Autodesk Fusion 360 part; units mm, degrees
note: some values were not read from the file. Chosen so that the rebuilt part matches the saved one: which bodies a step acts on. Set by a fixed rule: which sketch regions a step uses.
(part 2 of 2)
extrude "Extrude3" add sketch "Sketch1" along normal blind 6.7 contours L0 L1 L2 L3 L4 L5 A0 A1 A2 A3 A4 A5 bodies 1
extrude "Extrude5" add sketch "Sketch2" along normal blind 2 separate body contours A0 L0 L1 A80 A159 | A1 L2 L3 A80 A159 | A2 L4 L5 A81 A120 | A3 L6 L7 A81 A120 | A4 L8 L9 A82 A121 | A5 L10 L11 A82 A121 | A6 L12 L13 A83 A122 | A7 L14 L15 A83 A122 | A8 L16 L17 A84 A135 | A9 L18 L19 A84 A135 | A10 L20 L21 A85 A131 | A11 L22 L23 A85 A131 | A12 L24 L25 A86 A127 | A13 L26 L27 A86 A127 | A14 L28 L29 A87 A123 | A15 L30 L31 A87 A123 | A16 L32 L33 A88 A158 | A17 L34 L35 A88 A158 | A18 L36 L37 A89 A132 | A19 L38 L39 A89 A132 | A20 L40 L41 A90 A128 | A21 L42 L43 A90 A128 | A22 L44 L45 A91 A124 | A23 L46 L47 A91 A124 | A24 L48 L49 A92 A136 | A25 L50 L51 A92 A136 | A26 L52 L53 A93 A133 | A27 L54 L55 A93 A133 | A28 L56 L57 A94 A129 | A29 L58 L59 A94 A129 | A30 L60 L61 A95 A125 | A31 L62 L63 A95 A125 | A32 L64 L65 A96 A137 | A33 L66 L67 A96 A137 | A34 L68 L69 A97 A134 | A35 L70 L71 A97 A134 | A36 L72 L73 A98 A130 | A37 L74 L75 A98 A130 | A38 L76 L77 A99 A126 | A39 L78 L79 A99 A126 | A40 L80 L81 A100 A157 | A41 L82 L83 A100 A157 | A42 L84 L85 A101 A152 | A43 L86 L87 A101 A152 | A44 L88 L89 A102 A147 | A45 L90 L91 A102 A147 | A46 L92 L93 A103 A142 | A47 L94 L95 A103 A142 | A48 L96 L97 A104 A156 | A49 L98 L99 A104 A156 | A50 L100 L101 A105 A151 | A51 L102 L103 A105 A151 | A52 L104 L105 A106 A146 | A53 L106 L107 A106 A146 | A54 L108 L109 A107 A141 | A55 L110 L111 A107 A141 | A56 L112 L113 A108 A155 | A57 L114 L115 A108 A155 | A58 L116 L117 A109 A150 | A59 L118 L119 A109 A150 | A60 L120 L121 A110 A145 | A61 L122 L123 A110 A145 | A62 L124 L125 A111 A140 | A63 L126 L127 A111 A140 | A64 L128 L129 A112 A154 | A65 L130 L131 A112 A154 | A66 L132 L133 A113 A149 | A67 L134 L135 A113 A149 | A68 L136 L137 A114 A144 | A69 L138 L139 A114 A144 | A70 L140 L141 A115 A139 | A71 L142 L143 A115 A139 | A72 L144 L145 A116 A153 | A73 L146 L147 A116 A153 | A74 L148 L149 A117 A148 | A75 L150 L151 A117 A148 | A76 L152 L153 A118 A143 | A77 L154 L155 A118 A143 | A78 L156 L157 A119 A138 | A79 L158 L159 A119 A138 makes body 10 at (4.262, 7.3818, 0.6667) makes body 11 at (11.2811, -4.9625, 1.3333) makes body 12 at (-2.5256, 2.4663, 0.6667) makes body 13 at (12.115, 11.6015, 1.3333) makes body 14 at (22.5458, -5.5564, 0.6667) makes body 15 at (39.4227, -3.4161, 1.3333) makes body 16 at (33.1565, 1.6483, 1.3333) makes body 17 at (45.7149, 10.6668, 0.6667) makes body 18 at (16.2993, 19.8547, 1.3333) makes body 19 at (2.6839, 32.0105, 0.6667) makes body 20 at (27.8838, 27.9663, 1.3333) makes body 21 at (45.5449, 15.0482, 1.3333) makes body 22 at (12.7906, 14.4698, 1.3333) makes body 23 at (7.735, 27.078, 0.6667) makes body 24 at (21.9274, 24.1763, 1.3333) makes body 25 at (47.1273, 20.132, 0.6667) makes body 26 at (76.8247, -8.3362, 1.3333) makes body 27 at (96.5209, -4.8632, 1.3333) makes body 28 at (104.6325, 6.7213, 1.3333) makes body 29 at (84.0972, 9.8134, 1.3333) makes body 30 at (63.9057, 6.419, 1.3333) makes body 31 at (73.1464, 17.7127, 1.3333) makes body 32 at (89.7711, 21.0864, 1.3333) makes body 33 at (98.7218, 26.1059, 1.3333) makes body 34 at (80.6243, 29.5096, 1.3333) makes body 35 at (69.1776, 20.8965, 1.3333) makes body 36 at (71.4099, 27.5608, 1.3333) makes body 37 at (90.4723, 31.2461, 1.3333) makes body 38 at (101.0599, 23.2206, 1.3333) makes body 39 at (83.7119, 19.0225, 1.3333) makes body 40 at (62.6646, 16.1885, 1.3333) makes body 41 at (72.2711, 7.966, 1.3333) makes body 42 at (94.4246, 11.4019, 1.3333) makes body 43 at (106.369, -3.1267, 1.3333) makes body 44 at (86.6728, -6.5997, 1.3333) makes body 45 at (66.6168, -3.6556, 1.3333) makes body 46 at (32.8778, 27.3251, 1.3333) makes body 47 at (16.5459, 31.0086, 1.3333) makes body 48 at (4.4927, 23.0757, 1.3333) makes body 49 at (25.8487, 18.5212, 1.3333) makes body 50 at (17.5831, 25.3415, 0.6667) makes body 51 at (0.4947, 17.8012, 1.3333) makes body 52 at (22.1494, 12.8437, 1.3333) makes body 53 at (33.5476, 17.9766, 1.3333) makes body 54 at (41.3264, 6.4266, 1.3333) makes body 55 at (32.3297, -3.041, 1.3333) makes body 56 at (21.235, 2.8507, 1.3333) makes body 57 at (4.7147, 11.7431, 1.3333) makes body 58 at (8.415, 1.4895, 1.3333) makes body 59 at (2.1505, -2.7993, 1.3333) makes body 60 at (11.8885, 4.5947, 0.6667) makes body 61 at (18.2631, -0.2469, 1.3333) makes body 62 at (41.2681, -9.9363, 1.3333) makes body 63 at (32.7691, 7.8395, 1.3333) makes body 64 at (84.9363, 3.2484, 1.3333) makes body 65 at (65.2402, -0.2246, 1.3333) makes body 66 at (73.3518, 11.36, 1.3333) makes body 67 at (90.6102, 14.5214, 1.3333) makes body 68 at (100.3204, 32.9825, 1.3333) makes body 69 at (79.0256, 22.633, 1.3333) makes body 70 at (63.5191, 21.6152, 0.6667) makes body 71 at (42.0762, 25.0646, 0.6667) makes body 72 at (73.5479, -2.0827, 1.3333) makes body 73 at (93.244, 1.3903, 1.3333) makes body 74 at (101.3556, 12.9748, 1.3333) makes body 75 at (34.2958, 11.1964, 1.3333) makes body 76 at (41.0984, -0.6277, 1.3333) makes body 77 at (32.0698, -7.6757, 0.6667) makes body 78 at (19.9996, 9.6011, 1.3333) makes body 79 at (59.9311, 26.1228, 1.3333) makes body 80 at (91.3115, 24.681, 1.3333) makes body 81 at (100.4583, 16.2578, 1.3333) makes body 82 at (83.1999, 13.0965, 1.3333) makes body 83 at (58.9201, 10.8042, 0.6667) makes body 84 at (75.0883, 1.5119, 1.3333) makes body 85 at (94.7844, 4.9849, 1.3333) makes body 86 at (103.0921, 3.1267, 1.3333) makes body 87 at (83.396, -0.3462, 1.3333) makes body 88 at (66.9767, -10.0727, 1.3333) makes body 89 at (35.715, 20.9382, 1.3333)
extrude "Extrude7" add sketch "Sketch1" along normal blind 0.5 contours A18 L18 L19 A98 A154 | A19 L20 L21 A98 A154 | A20 L22 L23 A99 A155 | A21 L24 L25 A99 A155 | A22 L26 L27 A100 A156 | A23 L28 L29 A100 A156 | A24 L30 L31 A101 A157 | A25 L32 L33 A101 A157 | A26 L34 L35 A102 A161 | A27 L36 L37 A102 A161 | A28 L38 L39 A103 A160 | A29 L40 L41 A103 A160 | A30 L42 L43 A104 A159 | A31 L44 L45 A104 A159 | A32 L46 L47 A105 A158 | A33 L48 L49 A105 A158 | A34 L50 L51 A106 A162 | A35 L52 L53 A106 A162 | A36 L54 L55 A107 A163 | A37 L56 L57 A107 A163 | A38 L58 L59 A108 A164 | A39 L60 L61 A108 A164 | A40 L62 L63 A109 A165 | A41 L64 L65 A109 A165 | A42 L66 L67 A110 A169 | A43 L68 L69 A110 A169 | A44 L70 L71 A111 A168 | A45 L72 L73 A111 A168 | A46 L74 L75 A112 A167 | A47 L76 L77 A112 A167 | A48 L78 L79 A113 A166 | A49 L80 L81 A113 A166 | A50 L82 L83 A114 A170 | A51 L84 L85 A114 A170 | A52 L86 L87 A115 A171 | A53 L88 L89 A115 A171 | A54 L90 L91 A116 A172 | A55 L92 L93 A116 A172 | A56 L94 L95 A117 A173 | A57 L96 L97 A117 A173 | A58 L98 L99 A118 A193 | A59 L100 L101 A118 A193 | A60 L102 L103 A119 A192 | A61 L104 L105 A119 A192 | A62 L106 L107 A120 A191 | A63 L108 L109 A120 A191 | A64 L110 L111 A121 A190 | A65 L112 L113 A121 A190 | A66 L114 L115 A122 A186 | A67 L116 L117 A122 A186 | A68 L118 L119 A123 A187 | A69 L120 L121 A123 A187 | A70 L122 L123 A124 A188 | A71 L124 L125 A124 A188 | A72 L126 L127 A125 A189 | A73 L128 L129 A125 A189 | A74 L130 L131 A126 A185 | A75 L132 L133 A126 A185 | A76 L134 L135 A127 A184 | A77 L136 L137 A127 A184 | A78 L138 L139 A128 A183 | A79 L140 L141 A128 A183 | A80 L142 L143 A129 A182 | A81 L144 L145 A129 A182 | A82 L146 L147 A130 A178 | A83 L148 L149 A130 A178 | A84 L150 L151 A131 A179 | A85 L152 L153 A131 A179 | A86 L154 L155 A132 A180 | A87 L156 L157 A132 A180 | A88 L158 L159 A133 A181 | A89 L160 L161 A133 A181 | A90 L162 L163 A134 A177 | A91 L164 L165 A134 A177 | A92 L166 L167 A135 A176 | A93 L168 L169 A135 A176 | A94 L170 L171 A136 A175 | A95 L172 L173 A136 A175 | A96 L174 L175 A137 A174 | A97 L176 L177 A137 A174 bodies 1
extrude "Extrude6" add sketch "Sketch2" along normal blind 4 contours A80 A159 | A81 A120 | A82 A121 | A83 A122 | A84 A135 | A85 A131 | A86 A127 | A87 A123 | A88 A158 | A89 A132 | A90 A128 | A91 A124 | A92 A136 | A93 A133 | A94 A129 | A95 A125 | A96 A137 | A97 A134 | A98 A130 | A99 A126 | A100 A157 | A101 A152 | A102 A147 | A103 A142 | A104 A156 | A105 A151 | A106 A146 | A107 A141 | A108 A155 | A109 A150 | A110 A145 | A111 A140 | A112 A154 | A113 A149 | A114 A144 | A115 A139 | A116 A153 | A117 A148 | A118 A143 | A119 A138 bodies 80 81 82 83 84 85 86 87 88 89 50 51 52 59 60 61 62 63 35 75 76 77 78 10 11 17 18 19 20 71 72 73 74 64 65 66 67 68 69 70 12 14 79 53 54 55 56 57 58 13 15 16 21 22 23 24 25 26 27 28 29 30 31 32 33 34 36 37 38 39 40 41 42 43 44 45 46 47 48 49
sketch "Sketch4" plane through (0, 0, 6.7) normal (0, 0, 1) x (-1, 0, 0)
  line L0 (3.2654, 2.5) -> (101.4652, 2.5)
  line L1 (101.4652, 2.5) -> (101.4652, 6.7)
  line L2 (101.4652, 6.7) -> (3.2654, 6.7)
  line L3 (3.2654, 6.7) -> (3.2654, 2.5)
  arc A0 (-3.2654, -35.9157) -> (-0.3109, -33.4367) centre (-3.2654, -32.9157) ccw
  line L4 (-3.2654, -35.9157) -> (-101.4652, -35.9157)
  arc A1 (-104.4196, -33.4367) -> (-101.4652, -35.9157) centre (-101.4652, -32.9157) ccw
  line L5 (-104.4196, -33.4367) -> (-110.5811, 1.507)
  arc A2 (-108.1476, 4.9823) -> (-110.5811, 1.507) centre (-107.6267, 2.0279) ccw
  line L6 (-108.1476, 4.9823) -> (-61.1353, 13.2719)
  arc A3 (-60.6144, 13.3174) -> (-61.1353, 13.2719) centre (-60.6144, 10.3174) ccw
  line L7 (-60.6144, 13.3174) -> (-44.1162, 13.3174)
  arc A4 (-43.5952, 13.2719) -> (-44.1162, 13.3174) centre (-44.1162, 10.3174) ccw
  line L8 (-43.5952, 13.2719) -> (3.4171, 4.9823)
  arc A5 (5.8506, 1.507) -> (3.4171, 4.9823) centre (2.8961, 2.0279) ccw
  line L9 (5.8506, 1.507) -> (-0.3109, -33.4367)
  arc A6 (-2.0486, -37.6534) -> (0.9058, -35.1744) centre (-2.0486, -34.6534) ccw
  line L10 (0.9058, -35.1744) -> (7.5882, 2.7237)
  arc A7 (7.5882, 2.7237) -> (5.1548, 6.1991) centre (4.6338, 3.2446) ccw
  line L11 (5.1548, 6.1991) -> (-44.8119, 15.0095)
  arc A8 (-44.8119, 15.0095) -> (-45.3329, 15.0551) centre (-45.3329, 12.0551) ccw
  line L12 (-45.3329, 15.0551) -> (-59.3977, 15.0551)
  arc A9 (-59.3977, 15.0551) -> (-59.9186, 15.0095) centre (-59.3977, 12.0551) ccw
  line L13 (-59.9186, 15.0095) -> (-109.8853, 6.1991)
  arc A10 (-109.8853, 6.1991) -> (-112.3188, 2.7237) centre (-109.3644, 3.2446) ccw
  line L14 (-112.3188, 2.7237) -> (-105.6363, -35.1744)
  arc A11 (-105.6363, -35.1744) -> (-102.6819, -37.6534) centre (-102.6819, -34.6534) ccw
  line L15 (-102.6819, -37.6534) -> (-2.0486, -37.6534)
sketch "Sketch5" plane through (0, 0, 6.7) normal (0, 0, 1) x (-1, 0, 0)
  line L0 (-52.3653, -35.9157) -> (-58.3653, -35.9157)
  line L1 (-58.3653, -35.9157) -> (-58.3653, -37.6534)
  line L2 (-58.3653, -37.6534) -> (-52.3653, -37.6534)
  line L3 (-52.3653, -37.6534) -> (-52.3653, -35.9157)
  line L4 (-52.3653, -35.9157) -> (-46.3653, -35.9157)
  line L5 (-46.3653, -35.9157) -> (-46.3653, -37.6534)
  line L6 (-46.3653, -37.6534) -> (-52.3653, -37.6534)
  line L7 (-52.3653, -37.6534) -> (-52.3653, -35.9157)
  arc A0 (-3.2654, -35.9157) -> (-0.3109, -33.4367) centre (-3.2654, -32.9157) ccw
  line L8 (-3.2654, -35.9157) -> (-101.4652, -35.9157)
  arc A1 (-104.4196, -33.4367) -> (-101.4652, -35.9157) centre (-101.4652, -32.9157) ccw
  line L9 (-104.4196, -33.4367) -> (-110.5811, 1.507)
  arc A2 (-108.1476, 4.9823) -> (-110.5811, 1.507) centre (-107.6267, 2.0279) ccw
  line L10 (-108.1476, 4.9823) -> (-61.1353, 13.2719)
  arc A3 (-60.6144, 13.3174) -> (-61.1353, 13.2719) centre (-60.6144, 10.3174) ccw
  line L11 (-60.6144, 13.3174) -> (-44.1162, 13.3174)
  arc A4 (-43.5952, 13.2719) -> (-44.1162, 13.3174) centre (-44.1162, 10.3174) ccw
  line L12 (-43.5952, 13.2719) -> (3.4171, 4.9823)
  arc A5 (5.8506, 1.507) -> (3.4171, 4.9823) centre (2.8961, 2.0279) ccw
  line L13 (5.8506, 1.507) -> (-0.3109, -33.4367)
  arc A6 (-2.0486, -37.6534) -> (0.9058, -35.1744) centre (-2.0486, -34.6534) ccw
  line L14 (0.9058, -35.1744) -> (7.5882, 2.7237)
  arc A7 (7.5882, 2.7237) -> (5.1548, 6.1991) centre (4.6338, 3.2446) ccw
  line L15 (5.1548, 6.1991) -> (-44.8119, 15.0095)
  arc A8 (-44.8119, 15.0095) -> (-45.3329, 15.0551) centre (-45.3329, 12.0551) ccw
  line L16 (-45.3329, 15.0551) -> (-59.3977, 15.0551)
  arc A9 (-59.3977, 15.0551) -> (-59.9186, 15.0095) centre (-59.3977, 12.0551) ccw
  line L17 (-59.9186, 15.0095) -> (-109.8853, 6.1991)
  arc A10 (-109.8853, 6.1991) -> (-112.3188, 2.7237) centre (-109.3644, 3.2446) ccw
  line L18 (-112.3188, 2.7237) -> (-105.6363, -35.1744)
  arc A11 (-105.6363, -35.1744) -> (-102.6819, -37.6534) centre (-102.6819, -34.6534) ccw
  line L19 (-102.6819, -37.6534) -> (-2.0486, -37.6534)
  dimension "d35" = 6
  constraint horizontal L0
  constraint vertical L1
  constraint horizontal L2
  constraint vertical L3
  constraint horizontal L4
  constraint vertical L5
  constraint horizontal L6
  constraint vertical L7
  measures "d35" distance of L0.start L0.end
extrude "Extrude11" cut sketch "Sketch5" against normal blind 4.2 contours L0 L1 L2 L3 L7 L8 L19 | L3 L4 L5 L6 L7 L8 L19 bodies 1
fillet "Fillet1" radius 1.5 25 edges at (24.207, 37.6534, 6.7) (0.1203, 36.9516, 6.7) (-4.247, 16.2253, 6.7) (-7.0913, -4.9654, 6.7) (19.8286, -10.6043, 6.7) (45.0714, -15.0437, 6.7) (52.3653, -15.0551, 6.7) (59.6591, -15.0437, 6.7) (84.902, -10.6043, 6.7) (111.8218, -4.9654, 6.7) (108.9776, 16.2253, 6.7) (104.6103, 36.9516, 6.7) (80.5236, 37.6534, 6.7) (104.6103, 36.9516, 0) (108.9776, 16.2253, 0) (111.8218, -4.9654, 0) (84.902, -10.6043, 0) (59.6591, -15.0437, 0) (52.3653, -15.0551, 0) (45.0714, -15.0437, 0) (19.8286, -10.6043, 0) (-7.0913, -4.9654, 0) (-4.247, 16.2253, 0) (0.1203, 36.9516, 0) (52.3653, 37.6534, 0) on bodies 1
fillet "Fillet2" radius 1.2 40 edges at (-1.1071, 8.7452, 4) (7.0045, -2.8394, 4) (40.0217, 11.6473, 4) (10.4774, 16.8567, 4) (2.3658, 28.4413, 4) (22.062, 24.9683, 4) (67.1333, 23.2319, 4) (12.2139, 26.7048, 4) (0.6294, 18.5932, 4) (20.3255, 15.1203, 4) (-2.8436, -1.1029, 4) (8.741, 7.0087, 4) (16.8526, -4.5759, 4) (36.5487, -8.0489, 4) (28.4371, 3.5357, 4) (80.4543, 5.2722, 4) (60.7582, 1.7992, 4) (68.8698, 13.3838, 4) (88.5659, 16.8567, 4) (96.6775, 28.4413, 4) (76.9813, 24.9683, 4) (57.2852, 21.4954, 4) (41.7582, 21.4954, 4) (72.3427, -6.3124, 4) (92.0389, -2.8394, 4) (100.1505, 8.7452, 4) (30.1736, 13.3838, 4) (38.2852, 1.7992, 4) (26.7006, -6.3124, 4) (18.589, 5.2722, 4) (86.8294, 26.7048, 4) (98.414, 18.5932, 4) (78.7178, 15.1203, 4) (59.0217, 11.6473, 4) (70.6062, 3.5357, 4) (90.3024, 7.0087, 4) (101.8869, -1.1029, 4) (82.1908, -4.5759, 4) (62.4946, -8.0489, 4) (31.9101, 23.2319, 4) on bodies 10 11 17 18 19 20 35 50 51 52 59 60 61 62 63 64 65 66 67 68 69 70 71 72 73 74 75 76 77 78 80 81 82 83 84 85 86 87 88 89
fillet "Fillet3" radius 0.5 6 edges at (58.3653, 37.6534, 3.85) (58.3653, 37.2141, 6.2607) (58.3653, 36.0346, 6.7) (46.3653, 36.0346, 6.7) (46.3653, 37.2141, 6.2607) (46.3653, 37.6534, 3.85) on bodies 1
equation "plate_thickness = 2.5 mm"
equation "pole_height = 2.5 mm + plate_thickness + 0.1 mm" comment "reduced to 2.5mm (switch height)  + 0.1mm for tolerance. might be to low"
equation "wall_height = pole_height + pcb_thickness"
equation "pcb_thickness = 1.6 mm"
equation "d5 = plate_thickness"
equation "d7 = pole_height"
equation "d9 = wall_height"
equation "usb_cutout_length = 12 mm"
equation "key_base_thickness = 2 mm" comment "increased by 1"
equation "key_height = plate_thickness + 1.5 mm" comment "reduced by 1"
equation "d19 = key_base_thickness"
equation "d21 = key_height"
equation "key_rail_cutout_height = ( plate_thickness ) - key_base_thickness"
equation "d24 = key_rail_cutout_height"
equation "d35 = usb_cutout_length / 2"
equation "d36 = -wall_height + plate_thickness"
equation "case_walls_fillet = 1.5 mm"
equation "buttons_fillet = 1.2 mm"
equation "d45 = case_walls_fillet"
equation "d47 = buttons_fillet"
